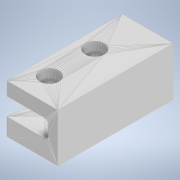
# Autodesk Inventor part: GlassesInterface
Saved by Autodesk Inventor 2020 (Build 240168000, 168)
## iProperties
Created: 2020-03-20
Part Number: GlassesInterface
Material: Generisch
Document SubType Name: Modeling
Designer: Fynn
Density: 1 g/cm^3
Appearance: Vorgabe
Author: Fynn
Autodesk Inventor part; units mm, degrees
ref_plane "YZ Plane" through (0, 0, 0) normal (1, 0, 0) x (0, 1, 0)
ref_plane "XZ Plane" through (0, 0, 0) normal (0, 1, 0) x (-1, 0, 0)
sketch "Skizze1" plane through (1.1129, -0.6689, -0.3576) normal (0, -1, 0) x (1, 0, 0)
  line L0 (0.75, -1.1424) -> (0.75, 1.8576) projected
  line L1 (0.75, 1.8576) -> (-0.58, 1.8576) projected
  line L2 (-0.58, 1.8576) -> (-0.58, -1.1424) projected
  line L3 (-0.58, -1.1424) -> (0.75, -1.1424) projected
  line L4 (0.75, 1.8576) -> (-0.58, 1.8576)
  line L5 (-0.58, 1.8576) -> (-0.58, -1.1424)
  line L6 (-0.58, -1.1424) -> (0.75, -1.1424)
  line L7 (0.75, -1.1424) -> (0.75, 1.8576)
  circle A0 centre (-0.15, 0) radius 0.25 projected
  circle A1 centre (-0.15, 0) radius 0.15 projected
  circle A2 centre (-0.13, 1.2) radius 0.15 projected
  circle A3 centre (-0.13, 1.2) radius 0.25 projected
  point P0 (-1.1129, 0.3576)
  constraints: 8 end point, 2 parallel, 1 horizontal, 1 perpendicular
sketch "Skizze2" plane through (0.5329, 0.5911, 1.5) normal (0, 0, 1) x (1, 0, 0)
  line L0 (0, -0.35) -> (1.0109, -0.35) projected
  circle A0 centre (0.98, -0.45) radius 0.1 projected
  line L1 (1.08, -0.4191) -> (1.08, -0.7409) projected
  circle A1 centre (0.98, -0.71) radius 0.1 projected
  line L2 (1.0109, -0.81) -> (0, -0.81) projected
  line L3 (1.33, -1.26) -> (1.33, 0) projected
  line L4 (1.33, 0) -> (0, 0) projected
  line L5 (1.33, -1.26) -> (0, -1.26) projected
  line L6 (0, -0.81) -> (0, -1.26) projected
  line L7 (0, 0) -> (0, -0.35) projected
  point P0 (-0.5329, -0.5911)
  point P1 (0.9799, -0.35)
  point P2 (1.08, -0.4499)
  point P3 (1.08, -0.7099)
  point P4 (0.9799, -0.81)
ref_plane "Arbeitsebene2" through (1.6129, -0.1189, -1.5) normal (0, 0, -1) x (-1, 0, 0)
extrude "Extrusion1" add sketch "Skizze2" against normal up to surface (3 mm away) contours L7 L4 L3 L5 L6 L2 A1 L1 A0 L0
extrude "Extrusion2" cut sketch "Skizze1" against normal blind 10 contours A1 | A2
sketch "Skizze3" plane through (0.5329, 0.5911, 1.5) normal (0, 1, 0) x (1, 0, 0)
  circle A0 centre (0.43, 1.8576) radius 0.15 projected
  circle A1 centre (0.45, 0.6577) radius 0.15 projected
  circle A2 centre (0.43, 1.8576) radius 0.2498
  circle A3 centre (0.45, 0.6577) radius 0.25
  point P0 (-0.5329, 1.5)
  dimension "d6" = 0.5
  constraints: 2 centre point, 2 coincident
  measures "d6" diameter of A3
extrude "Extrusion3" cut sketch "Skizze3" against normal blind 0.25
